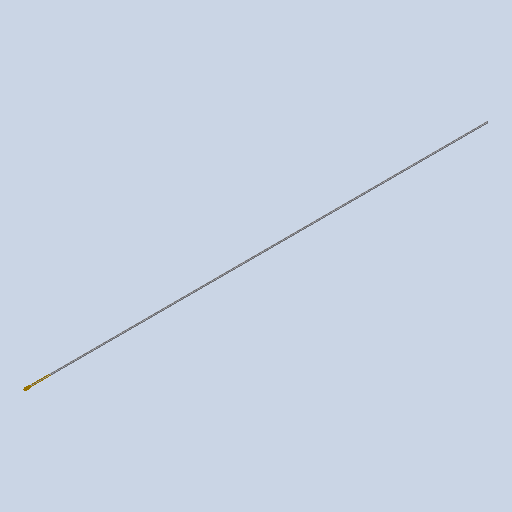
# Autodesk Inventor part: 13-106
Saved by Autodesk Inventor 2022 (Build 260153000, 153)
## iProperties
Created: 2004-09-17
Part Number: 13-106
Material: Alluminio - 6061
Document SubType Name: Modeling
Designer: Chapin
Manufacturer: Standard
Standards Organization: Custom
Mass: 24.2961 g
Surface Area: 156.08 cm^2
Volume: 8.96535 cm^3
Density: 2.71 g/cm^3
Appearance: Alluminio - Piatto
d30: 0,000 mm
d34: 0,000 mm
d35: 0,000 mm
d36: 0,000 mm
d38: 0,000 mm
d39: 0,000 mm
Author: Chapin
Autodesk Inventor part; units mm, degrees
ref_plane "YZ Plane" through (0, 0, 0) normal (1, 0, 0) x (0, 1, 0)
ref_plane "XY Plane" through (0, 0, 0) normal (0, 0, 1) x (1, 0, 0)
sketch "Sketch1" plane through (0, 0, 0) normal (0, 0, 1) x (1, 0, 0)
  line L0 (-6.5, 5.5) -> (6.5, 5.5)
  line L1 (6.5, 5.5) -> (6.5, -5.5)
  line L2 (6.5, -5.5) -> (-6.5, -5.5)
  line L3 (-6.5, -5.5) -> (-6.5, 5.5)
  point P0 (0, 0)
  dimension "d0" = 13
  dimension "d1" = 11
  dimension "d2" = 6.5
  dimension "d3" = 5.5
  constraints: 8 end point, 2 parallel, 1 horizontal, 1 perpendicular
  measures "d0" distance of L0.start L0.end
  measures "d1" distance of L2.end L0.start
  measures "d2" distance from line of point (0, 0) L3
  measures "d3" distance from line of point (0, 0) L0
extrude "Extrusion1" add sketch "Sketch1" against normal blind 4000
sketch "Sketch2" plane through (0, 0, 0) normal (0, 0, 1) x (1, 0, 0)
  line L0 (-6.5, 5.5) -> (6.5, 5.5) projected
  line L1 (-6.5, -5.5) -> (-6.5, 5.5) projected
  line L2 (6.5, -5.5) -> (-6.5, -5.5) projected
  line L3 (6.5, 5.5) -> (6.5, -5.5) projected
  line L4 (-6.5, 4.5) -> (-4.2125, 4.5)
  line L5 (-4.2125, 4.5) -> (-4.2125, -0.1875)
  line L6 (-4.2125, -0.1875) -> (-4, -0.4)
  line L7 (-4, -0.4) -> (-4, -5.5)
  line L8 (0, 7.7) -> (0, -7.7) projected
  line L9 (-6.5, 4.5) -> (-6.5, -5.5)
  line L10 (-6.5, -5.5) -> (-4, -5.5)
  dimension "d6" = 1
  dimension "d7" = 8.425
  dimension "d8" = 8
  dimension "d9" = 135
  dimension "d10" = 5.1
  constraints: 12 end point, 3 perpendicular, 2 collinear, 2 point on line
  measures "d6" distance between parallel lines of L0 L4
  measures "d7" diameter of L5 L8
  measures "d8" diameter of L7 L8
  measures "d9" angle of L7 L6
  measures "d10" distance of L6.end L7.end
extrude "Extrusion2" cut sketch "Sketch2" against normal through all contours L4 L5 L6 L7 L2 L1
fillet "Fillet1" radius 1 1 edges at (-4.2125, 4.5, -2000)
fillet "Fillet1" radius 1.1 1 edges at (-4, -5.5, -2000)
mirror "Mirror1" about plane through (0, 0, 0) normal (1, 0, 0) of "Extrusion2", "Fillet1"
sketch "Sketch3" plane through (0, 0, 0) normal (0, 0, 1) x (1, 0, 0)
  line L0 (-6.5, 5.5) -> (6.5, 5.5) projected
  line L1 (-4.2125, 3.5) -> (-4.2125, -0.1875) projected
  line L2 (-4.2125, -0.1875) -> (-4, -0.4) projected
  line L3 (-4, -0.4) -> (-4, -4.4) projected
  line L4 (2.9, -5.5) -> (-2.9, -5.5) projected
  arc A0 (-3.05, 5.1) -> (-3.05, 5.5) centre (-3.05, 5.3) ccw
  line L5 (-3.1625, 0.2474) -> (-2.95, 0.0349)
  line L6 (-2.95, 0.0349) -> (-2.95, -4.46)
  line L7 (-2.95, -4.46) -> (-0.9867, -4.46)
  line L8 (0, 7.7) -> (0, -7.7) projected
  line L9 (-3.1625, 0.2474) -> (-3.1625, 5.1)
  line L10 (-3.05, 5.1) -> (-3.1625, 5.1)
  line L11 (-0.775, 1.6018) -> (-0.9867, -4.46)
  line L12 (0, 1.5) -> (0, -5.5)
  arc A1 (-0.775, 1.6018) -> (0, 1.5) centre (0, 4.5) ccw
  line L13 (0, 1.5) -> (0, 5.5)
  line L14 (0, 5.5) -> (-3.05, 5.5)
  dimension "d15" = 0.4
  dimension "d16" = 1
  dimension "d18" = 5.7
  dimension "d19" = 1.05
  dimension "d20" = 1.05
  dimension "d21" = 1.05
  dimension "d22" = 92
  dimension "d23" = 1.04
  dimension "d24" = 1.55
  dimension "d25" = 3
  constraints: 18 end point, 5 point on line, 4 point on circle, 3 parallel, 2 centre point, 2 midpoint, 2 perpendicular, 2 tangent, 1 coincident
  measures "d15" diameter of A0
  measures "d16" distance from line of L0 point (0, 4.5)
  measures "d19" distance between parallel lines of L9 L1
  measures "d20" distance between parallel lines of L5 L2
  measures "d21" distance between parallel lines of L3 L6
  measures "d22" angle of L7 L11
  measures "d23" distance between parallel lines of L4 L7
  measures "d24" diameter of L11.start L8
  measures "d25" radius of A1
extrude "Extrusion3" cut sketch "Sketch3" against normal through all
mirror "Mirror2" about plane through (0, 0, 0) normal (1, 0, 0) of "Extrusion3"
fillet "Fillet2" radius 0.4 4 edges at (-2.95, -4.46, -2000) (-0.9867, -4.46, -2000) (0.9867, -4.46, -2000) (2.95, -4.46, -2000)
ref_plane "Side1" through (-6.5, 4.5, 0) normal (0, -1, 0) x (1, 0, 0)
ref_plane "T-Slot1" through (0, 5.5, 0) normal (1, 0, 0) x (0, 0, -1)
ref_plane "Side3" through (-6.5, 5.5, 0) normal (0, 1, 0) x (-1, 0, 0)
ref_plane "Side2" through (6.5, 5.5, 0) normal (1, 0, 0) x (0, 1, 0)
ref_plane "Piano di lavoro5" through (0, 1.5, 0) normal (0, 1, 0) x (-1, 0, 0)
equation "\"d2\" = 0.5 * d0"
equation "\"d3\" = 0.5 * d1"
equation "\"d4\" = Ex_Length"
equation "\"Ex_Length\" = 4000"
